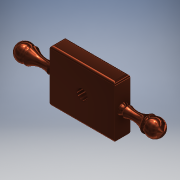
# Autodesk Inventor part: Guard
Saved by Autodesk Inventor 2017 (Build 210142000, 142)
## iProperties
Created: 2019-06-22
Part Number: Guard
Material: Copper
Document SubType Name: Modeling
Designer: Ole Simmering
Density: 8.94 g/cm^3
Appearance: Copper - Polished
Author: Ole Simmering
Autodesk Inventor part; units mm, degrees
ref_plane "YZ Plane" through (0, 0, 0) normal (1, 0, 0) x (0, 1, 0)
ref_plane "XZ Plane" through (0, 0, 0) normal (0, 1, 0) x (-1, 0, 0)
ref_plane "XY Plane" through (0, 0, 0) normal (0, 0, 1) x (1, 0, 0)
sketch "Sketch1" plane through (0, 0, 0) normal (0, 0, 1) x (1, 0, 0)
  line L0 (0, 0) -> (-25, 0)
  line L1 (-25, 0) -> (-25, 6)
  line L2 (-25, 6) -> (0, 6)
  line L3 (0, 6) -> (0, 0)
  dimension "d0" = 6
  dimension "d1" = 25
  constraints: 8 end point, 2 parallel, 1 horizontal, 1 perpendicular
  measures "d0" distance of L2.end L0.start
  measures "d1" distance of L1.end L2.end
extrude "Extrusion1" add sketch "Sketch1" along normal blind 20
ref_plane "Work Plane3" through (-25, 3, 0) normal (0, 1, 0) x (1, 0, 0)
sketch "Sketch4" plane through (-25, 3, 0) normal (0, 1, 0) x (1, 0, 0)
  line L0 (25, 0) -> (25, -20) construction
  line L1 (25, -10) -> (37.1082, -10) construction
  line L2 (25, -10) -> (25, -12)
  arc A0 (34.75, -13) -> (27, -12) centre (29.9371, -19.7686) ccw
  line L3 (34.75, -13) -> (34.75, -12.5)
  line L4 (34.75, -12.5) -> (34.9, -12.5)
  line L5 (34.9, -12.5) -> (34.95, -13)
  line L6 (35, -13.5) -> (35.05, -13) construction
  arc A1 (36.2518, -13) -> (35.1, -12.5) centre (35.1, -14.0767) ccw
  arc A2 (27, -12) -> (25, -12) centre (26, -13.118) ccw
  line L7 (27, -12) -> (25, -12) construction
  line L8 (34.75, -13) -> (35.25, -13) construction
  line L9 (35, -13.5) -> (35, -12.5526) construction
  line L10 (34.9, -12.5) -> (23.9137, -12.5) construction
  arc A3 (36.2518, -13) -> (40.001, -12) centre (37.4596, -10) ccw
  line L11 (40.001, -12) -> (40.7289, -10)
  line L12 (25, -10) -> (40.7289, -10)
  line L13 (34.95, -13) -> (35.05, -13)
  line L14 (34.95, -13) -> (35, -13.5) construction
  line L15 (35.05, -13) -> (35.1, -12.5)
  line L16 (35.1, -12.5) -> (35.1, -36.5539) construction
  dimension "d5" = 5
  dimension "d6" = 6
  dimension "d9" = 2
  dimension "d10" = 1.5
  dimension "d11" = 9.75
  dimension "d13" = 4
  dimension "d14" = 10
  dimension "d15" = 0.2
  dimension "d20" = 70
  dimension "d21" = 4
  dimension "d23" = 7
  dimension "d24" = 6
  constraints: 32 end point, 9 point on circle, 4 centre point, 4 point on line, 4 vertical, 3 horizontal, 2 line through centre, 1 collinear, 1 midpoint, 1 perpendicular, 1 tangent, 2 other
  measures "d5" diameter of L4 L1
  measures "d6" diameter of L3.start L1
  measures "d9" distance from line of L0 L7.start
  measures "d10" radius of A2
  measures "d11" distance from line of L3.start L0
  measures "d13" diameter of L2.end L1
  measures "d14" distance from line of L0 L6.start
  measures "d15" distance of L4.end L15.end
  measures "d20" angle of L1 L11
  measures "d21" diameter of L11.start L1
  measures "d23" diameter of L6.start L1
  measures "d24" diameter of A1.start L1
revolve "Revolution1" add sketch "Sketch4" angle 360 about axis through (0, 3, 10) along (1, 0, 0)
ref_plane "Work Plane4" through (-12.5, 0, 20) normal (1, 0, 0) x (0, 0, -1)
mirror "Mirror1" about plane through (-12.5, 0, 20) normal (1, 0, 0) of "Revolution1"
fillet "Fillet1" radius 1 8 edges at (-25, 3, 20) (-12.5, 6, 20) (-12.5, 0, 20) (0, 3, 20) (-12.5, 6, 0) (-25, 3, 0) (-12.5, 0, 0) (0, 3, 0)
fillet "Fillet2" radius 0.1 12 edges at (-0.2929, 5.7071, 19.7071) (0, 6, 10) (-0.2929, 0.2929, 19.7071) (0, 0, 10) (-0.2929, 5.7071, 0.2929) (-0.2929, 0.2929, 0.2929) (-24.7071, 0.2929, 0.2929) (-25, 0, 10) (-24.7071, 0.2929, 19.7071) (-24.7071, 5.7071, 19.7071) (-25, 6, 10) (-24.7071, 5.7071, 0.2929)
sketch "Sketch5" plane through (-15.9, 6, 19) normal (0, 1, 0) x (1, 0, 0)
  line L0 (-9, 0) -> (-9, 18) construction
  line L1 (15.8, 0) -> (-9, 0) construction
  line L2 (15.8, 18) -> (15.8, 0) construction
  line L3 (-9, 18) -> (15.8, 18) construction
  point P0 (3.4, 9)
hole "Hole1" at (-12.5, 6, 10) direction (0, -1, 0) diameter 4 end through all
body "Solid1"
